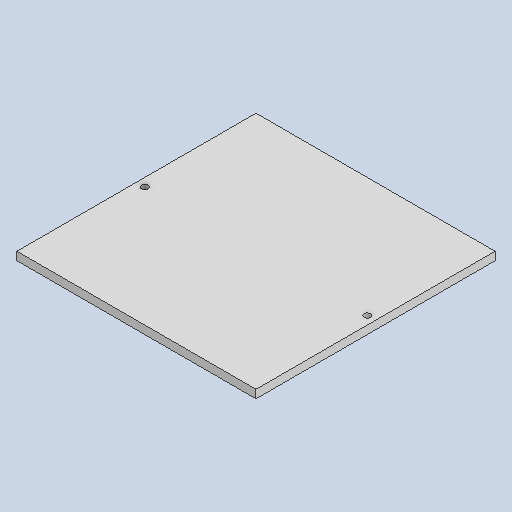
# Autodesk Inventor part: pot_mover
Saved by Autodesk Inventor 2023 (Build 270158000, 158)
## iProperties
Created: 2022-06-26
Part Number: pot_mover
Material: Generic
Document SubType Name: Modeling
Designer: prana_p9lsmih
Density: 1 g/cm^3
Appearance: Default
Author: prana_p9lsmih
Autodesk Inventor part; units mm, degrees
ref_plane "YZ Plane" through (0, 0, 0) normal (1, 0, 0) x (0, 1, 0)
ref_plane "XZ Plane" through (0, 0, 0) normal (0, 1, 0) x (-1, 0, 0)
ref_plane "XY Plane" through (0, 0, 0) normal (0, 0, 1) x (1, 0, 0)
sketch "Sketch1" plane through (0, 0, 0) normal (0, 1, 0) x (-1, 0, 0)
  line L0 (0, 0) -> (145, 0)
  line L1 (145, 0) -> (145, -145)
  line L2 (145, -145) -> (0, -145)
  line L3 (0, -145) -> (0, 0)
  dimension "d0" = 145
  dimension "d1" = 145
  constraints: 8 end point, 2 parallel, 1 horizontal, 1 perpendicular
  measures "d0" distance of L1.end L2.end
  measures "d1" distance of L0.end L1.end
extrude "Extrusion1" add sketch "Sketch1" along normal blind 5
sketch "Sketch2" plane through (0, 5, 0) normal (0, 1, 0) x (1, 0, 0)
  line L0 (-145, 145) -> (-145, 0) projected
  line L1 (0, 145) -> (-145, 145) projected
  point P0 (0, 0)
  point P1 (-140, 72.5)
  dimension "d4" = 5
  dimension "d5" = 72.5
  measures "d4" distance from line of L0 point (-140, 72.5)
  measures "d5" distance from line of L1 point (-140, 72.5)
hole "Hole1" at (-140, 5, -72.5) direction (0, -1, 0) diameter 4 end through all
sketch "Sketch3" plane through (0, 5, 0) normal (0, 1, 0) x (1, 0, 0)
  line L0 (0, 0) -> (0, 145) projected
  line L1 (0, 145) -> (-145, 145) projected
  point P0 (-5, 72.5)
  dimension "d13" = 5
  dimension "d14" = 72.5
  measures "d13" distance from line of L0 point (-5, 72.5)
  measures "d14" distance from line of L1 point (-5, 72.5)
hole "Hole2" at (-5, 5, -72.5) direction (0, -1, 0) diameter 4 end through all
body "Solid1"
